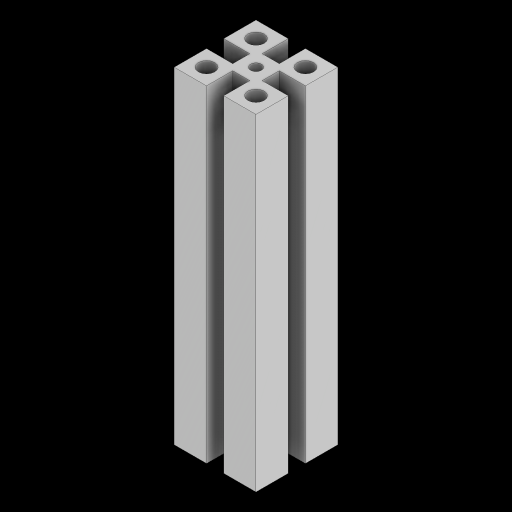
# Autodesk Inventor part: 3030column
Saved by Autodesk Inventor 2023 (Build 270158000, 158)
## iProperties
Created: 2024-07-03
Part Number: 3030column
Material: 일반
Document SubType Name: Modeling
Designer: OMS55
Density: 1 g/cm^3
Appearance: 기본값
Author: OMS55
Autodesk Inventor part; units mm, degrees
ref_plane "YZ Plane" through (0, 0, 0) normal (1, 0, 0) x (0, 1, 0)
ref_plane "XZ Plane" through (0, 0, 0) normal (0, 1, 0) x (-1, 0, 0)
ref_plane "XY Plane" through (0, 0, 0) normal (0, 0, 1) x (1, 0, 0)
sketch "스케치1" plane through (0, 0, 0) normal (0, 1, 0) x (-1, 0, 0)
  line L0 (0, 0) -> (-30, 0)
  line L1 (-30, 0) -> (-30, -30)
  line L2 (-30, -30) -> (0, -30)
  line L3 (0, -30) -> (0, 0)
  dimension "d0" = 30
  dimension "d1" = 30
  constraints: 8 end point, 2 parallel, 1 coincident, 1 horizontal, 1 perpendicular
  measures "d0" distance of L2.end L0.start
  measures "d1" distance of L1.end L2.end
extrude "돌출1" add sketch "스케치1" along normal blind 120
sketch "스케치6" plane through (0, 120, 0) normal (0, 1, 0) x (1, 0, 0)
  line L0 (0, 11.85) -> (9.6, 11.85)
  line L1 (9.6, 11.85) -> (9.6, 18.15)
  line L2 (9.6, 18.15) -> (0, 18.15)
  line L3 (0, 18.15) -> (0, 11.85)
  line L4 (0, 30) -> (0, 0) projected
  line L5 (0, 0) -> (30, 0) construction
  line L6 (15, 0) -> (15, 30) construction
  line L7 (30, 30) -> (0, 30) construction
  line L8 (0, 15) -> (30, 15) construction
  line L9 (11.85, 0) -> (18.15, 0)
  line L10 (18.15, 0) -> (18.15, 9.6)
  line L11 (18.15, 9.6) -> (11.85, 9.6)
  line L12 (11.85, 9.6) -> (11.85, 0)
  line L13 (0, 30) -> (30, 30) construction
  line L14 (11.85, 30) -> (18.15, 30)
  line L15 (18.15, 30) -> (18.15, 20.4)
  line L16 (18.15, 20.4) -> (11.85, 20.4)
  line L17 (11.85, 20.4) -> (11.85, 30)
  line L18 (30, 11.85) -> (20.4, 11.85)
  line L19 (20.4, 11.85) -> (20.4, 18.15)
  line L20 (20.4, 18.15) -> (30, 18.15)
  line L21 (30, 18.15) -> (30, 11.85)
  dimension "d15" = 6.3
  dimension "d16" = 9.6
  dimension "d17" = 9.6
  dimension "d18" = 6.3
  constraints: 38 end point, 8 symmetric about line, 6 midpoint, 4 parallel, 3 horizontal, 2 perpendicular
  measures "d15" distance of L2.end L0.start
  measures "d16" distance of L1.end L2.end
  measures "d17" distance of L11.end L9.start
  measures "d18" distance of L9.start L9.end
extrude "돌출4" cut sketch "스케치6" against normal blind 500
sketch "스케치7" plane through (0, 120, 0) normal (0, 1, 0) x (1, 0, 0)
  circle A0 centre (5.925, 5.925) radius 3
  circle A1 centre (5.925, 24.075) radius 3
  circle A2 centre (24.075, 24.075) radius 3
  circle A3 centre (24.075, 5.925) radius 3
  circle A4 centre (15, 15) radius 2
  line L0 (0, 0) -> (11.85, 0) projected
  line L1 (0, 11.85) -> (0, 0) projected
  line L2 (11.85, 30) -> (0, 30) projected
  line L3 (30, 18.15) -> (30, 30) projected
  line L4 (9.6, 18.15) -> (9.6, 11.85) projected
  line L5 (18.15, 20.4) -> (11.85, 20.4) projected
  point P0 (9.6, 15)
  point P1 (15, 20.4)
  dimension "d21" = 6
  dimension "d22" = 6
  dimension "d23" = 6
  dimension "d24" = 6
  dimension "d25" = 5.925
  dimension "d26" = 5.925
  dimension "d27" = 5.925
  dimension "d28" = 5.925
  dimension "d29" = 4
  constraints: 5 centre point, 3 horizontal alignment, 3 vertical alignment, 2 midpoint
  measures "d21" diameter of A0
  measures "d22" diameter of A1
  measures "d23" diameter of A2
  measures "d24" diameter of A3
  measures "d25" distance from line of L0 A0.centre
  measures "d26" distance from line of L1 A0.centre
  measures "d27" distance from line of L2 A1.centre
  measures "d28" distance from line of L3 A2.centre
  measures "d29" diameter of A4
extrude "돌출5" cut sketch "스케치7" against normal blind 200
